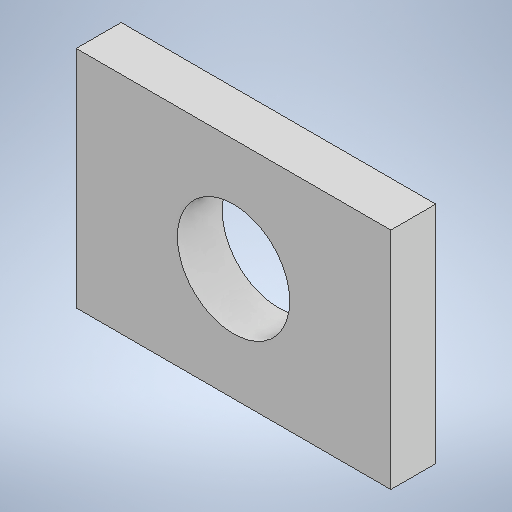
# Autodesk Inventor part: rama_1
Saved by Autodesk Inventor 2025.2 (Build 292293000, 293)
## iProperties
Created: 2025-04-28
Part Number: rama_1
Material: Ogólny
Document SubType Name: Modeling
Designer: marci
Density: 1 g/cm^3
Appearance: Domyślna
Author: marci
Autodesk Inventor part; units mm, degrees
ref_plane "YZ Plane" through (0, 0, 0) normal (1, 0, 0) x (0, 1, 0)
ref_plane "XZ Plane" through (0, 0, 0) normal (0, 1, 0) x (-1, 0, 0)
ref_plane "XY Plane" through (0, 0, 0) normal (0, 0, 1) x (1, 0, 0)
sketch "Szkic1" plane through (0, 0, 0) normal (0, 0, 1) x (1, 0, 0)
  circle A0 centre (0, 0) radius 12.5
  line L0 (35, 25) -> (-35, 25)
  line L1 (-35, 25) -> (-35, -25)
  line L2 (-35, -25) -> (35, -25)
  line L3 (35, -25) -> (35, 25)
  dimension "d0" = 25
  dimension "d1" = 70
  dimension "d2" = 50
  constraints: 8 end point, 2 parallel, 1 centre point, 1 coincident, 1 horizontal, 1 perpendicular
  measures "d0" diameter of A0
  measures "d1" distance of L2.end L1.end
  measures "d2" distance of L1.end L0.end
extrude "Wyciągnięcie proste1" add sketch "Szkic1" along normal blind 10
